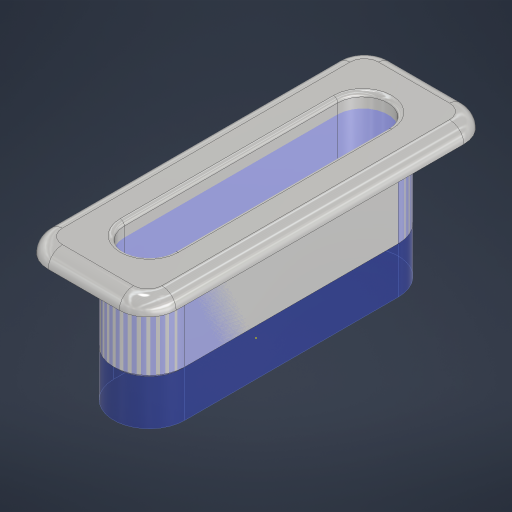
# Autodesk Inventor part: Aisle L40
Saved by Autodesk Inventor 2024.3 (Build 283343000, 343)
## iProperties
Created: 2021-09-15
Part Number: Aisle L40
Material: Aluminum 6061-AHC
Document SubType Name: Modeling
Designer: sauliusd
Density: 2.7 g/cm^3
Appearance: Aluminum - Dark
Length: 40,000 mm
Author: sauliusd
Autodesk Inventor part; units mm, degrees
ref_plane "YZ Plane" through (0, 0, 0) normal (1, 0, 0) x (0, 1, 0)
ref_plane "XZ Plane" through (0, 0, 0) normal (0, 1, 0) x (-1, 0, 0)
ref_plane "XY Plane" through (0, 0, 0) normal (0, 0, 1) x (1, 0, 0)
sketch "Sketch1" plane through (0, 0, 0) normal (0, 0, 1) x (1, 0, 0)
  line L0 (-15, 0) -> (15, 0) construction
  line L1 (-15, -5) -> (15, -5)
  line L2 (15, 5) -> (-15, 5)
  arc A0 (-15, 5) -> (-15, -5) centre (-15, 0) ccw
  arc A1 (15, -5) -> (15, 5) centre (15, 0) ccw
  line L3 (-20, -5) -> (20, -5) construction
  line L4 (20, -5) -> (20, 5) construction
  line L5 (20, 5) -> (-20, 5) construction
  line L6 (-20, 5) -> (-20, -5) construction
  line L7 (-20, -5) -> (20, 5) construction
  line L8 (20, -5) -> (-20, 5) construction
  point P0 (0, 0)
  dimension "d1" = 10
  dimension "Length" = 40
  constraints: 20 end point, 5 tangent, 4 point on circle, 3 midpoint, 3 parallel, 2 centre point, 2 horizontal, 1 collinear, 1 perpendicular
  measures "d1" diameter of A1
  measures "Length" distance of L4.end L5.end
extrude "Extrusion1" add sketch "Sketch1" against normal blind 18
sketch "Sketch2" plane through (0, 0, 0) normal (0, 0, 1) x (1, 0, 0)
  line L0 (-24.2177, -9) -> (24.2177, -9)
  line L1 (24.2177, -9) -> (24.2177, 9)
  line L2 (24.2177, 9) -> (-24.2177, 9)
  line L3 (-24.2177, 9) -> (-24.2177, -9)
  line L4 (-24.2177, -9) -> (24.2177, 9) construction
  line L5 (24.2177, -9) -> (-24.2177, 9) construction
  line L6 (15, 5) -> (-15, 5) projected
  line L7 (-20, 5.8694) -> (-20, -5.995) construction
  arc A0 (-15, 5) -> (-15, -5) centre (-15, 0) ccw projected
  point P0 (0, 0)
  dimension "d4" = 4
  dimension "d5" = 4.2177
  constraints: 14 end point, 2 midpoint, 2 parallel, 1 horizontal, 1 perpendicular, 1 tangent, 1 vertical
  measures "d4" distance between parallel lines of L6 L2
  measures "d5" distance between parallel lines of L3 L7
extrude "Extrusion2" add sketch "Sketch2" along normal blind 2 separate body
sketch "Sketch3" plane through (0, 0, 0) normal (0, 0, -1) x (-1, 0, 0)
  arc A0 (-15, 5) -> (-15, -5) centre (-15, 0) ccw projected
  line L0 (-15, -5) -> (15, -5) projected
  arc A1 (15, -5) -> (15, 5) centre (15, 0) ccw projected
  line L1 (15, 5) -> (-15, 5) projected
  point P0 (0, 0)
extrude "Extrusion3" add sketch "Sketch3" along normal blind 12 bodies 2
sketch "Sketch4" plane through (0, 0, -12) normal (0, 0, -1) x (-1, 0, 0)
  line L0 (-15, -5) -> (15, -5) projected
  arc A0 (15, -5) -> (15, 5) centre (15, 0) ccw projected
  line L1 (15, 5) -> (-15, 5) projected
  arc A1 (-15, 5) -> (-15, -5) centre (-15, 0) ccw projected
  line L2 (15, -3.5) -> (-15, -3.5)
  arc A2 (-15, 3.5) -> (-15, -3.5) centre (-15, 0) ccw
  line L3 (-15, 3.5) -> (15, 3.5)
  arc A3 (15, -3.5) -> (15, 3.5) centre (15, 0) ccw
  point P0 (0, 0)
  dimension "d10" = 1.5
  constraints: 4 end point, 4 point on circle, 2 centre point, 3 other
  measures "d10" distance between parallel lines of L0 L2
extrude "Extrusion4" cut sketch "Sketch4" against normal through all contours L2 A2 L3 A3 bodies 2
fillet "Fillet1" radius 4 4 edges at (-24.2177, -9, 1) (-24.2177, 9, 1) (24.2177, -9, 1) (24.2177, 9, 1)
fillet "Fillet2" radius 2 8 edges at (-23.0462, -7.8284, 2) (0, -9, 2) (23.0462, -7.8284, 2) (24.2177, 0, 2) (23.0462, 7.8284, 2) (0, 9, 2) (-23.0462, 7.8284, 2) (-24.2177, 0, 2)
fillet "Fillet3" radius 0.6 4 edges at (18.5, 0, 2) (0, -3.5, 2) (-18.5, 0, 2) (0, 3.5, 2)
chamfer "Chamfer1" distance 0.5 angle 45 4 edges at (0, -5, -12) (-20, 0, -12) (0, 5, -12) (20, 0, -12)
sketch "Sketch5" plane through (0, 0, -18) normal (0, 0, -1) x (-1, 0, 0)
  point P0 (0, 0)
body "Solid2"
